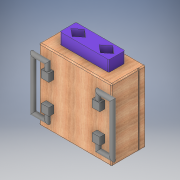
# Autodesk Inventor part: T9 Middle
Saved by Autodesk Inventor 2018 (Build 220112000, 112)
## iProperties
Created: 2018-02-18
Part Number: T9 Middle
Material: Wood (Birch)
Document SubType Name: Modeling
Designer: Blue Mist
Density: 0.55 g/cm^3
Appearance: Birch - Natural Polished
Author: Blue Mist
Autodesk Inventor part; units mm, degrees
ref_plane "YZ Plane" through (0, 0, 0) normal (1, 0, 0) x (0, 1, 0)
ref_plane "XZ Plane" through (0, 0, 0) normal (0, 1, 0) x (-1, 0, 0)
ref_plane "XY Plane" through (0, 0, 0) normal (0, 0, 1) x (1, 0, 0)
sketch "Sketch1" plane through (0, 0, 0) normal (0, 0, 1) x (1, 0, 0)
  line L0 (1.27, 0) -> (80.772, 0)
  line L1 (82.042, 1.27) -> (82.042, 79.375)
  line L2 (80.772, 80.645) -> (1.27, 80.645)
  line L3 (0, 79.375) -> (0, 1.27)
  arc A0 (82.042, 79.375) -> (80.772, 80.645) centre (80.772, 79.375) ccw
  arc A1 (80.772, 0) -> (82.042, 1.27) centre (80.772, 1.27) ccw
  arc A2 (0, 1.27) -> (1.27, 0) centre (1.27, 1.27) ccw
  arc A3 (1.27, 80.645) -> (0, 79.375) centre (1.27, 79.375) ccw
  point P0 (0, 0)
  point P1 (82.042, 80.645)
  point P2 (82.042, 0)
  point P3 (0, 80.645)
  dimension "d0" = 82.042
  dimension "d1" = 80.645
  dimension "d2" = 1.27
  constraints: 8 end point, 8 point on circle, 8 point on line, 8 tangent, 4 centre point, 3 equal radius, 2 parallel, 1 horizontal, 1 perpendicular
  measures "d0" distance of point (0, 80.645) point (82.042, 80.645)
  measures "d1" distance of point (82.042, 80.645) point (82.042, 0)
  measures "d2" radius of A0
extrude "Extrusion1" add sketch "Sketch1" against normal blind 38.5318
sketch "Sketch2" plane through (0, 0, -38.5318) normal (0, 0, -1) x (-1, 0, 0)
  line L0 (-80.772, 0) -> (-1.27, 0) projected
  line L1 (-1.27, 80.645) -> (-80.772, 80.645) projected
  line L2 (0, 1.27) -> (0, 79.375) construction
  line L3 (-82.042, 79.375) -> (-82.042, 1.27) construction
  line L4 (-63.119, 20.8915) -> (-18.923, 20.8915)
  line L5 (-17.653, 22.1615) -> (-17.653, 58.4835)
  line L6 (-18.923, 59.7535) -> (-63.119, 59.7535)
  line L7 (-64.389, 58.4835) -> (-64.389, 22.1615)
  arc A0 (-64.389, 22.1615) -> (-63.119, 20.8915) centre (-63.119, 22.1615) ccw
  arc A1 (-18.923, 20.8915) -> (-17.653, 22.1615) centre (-18.923, 22.1615) ccw
  arc A2 (-17.653, 58.4835) -> (-18.923, 59.7535) centre (-18.923, 58.4835) ccw
  arc A3 (-63.119, 59.7535) -> (-64.389, 58.4835) centre (-63.119, 58.4835) ccw
  point P0 (0, 0)
  point P1 (-64.389, 20.8915)
  point P2 (-17.653, 59.7535)
  dimension "d5" = 80.645
  dimension "d8" = 82.042
  dimension "d9" = 17.653
  dimension "d10" = 20.8915
  dimension "d11" = 20.8915
  dimension "d12" = 17.653
  dimension "d13" = 1.27
  constraints: 8 end point, 8 point on circle, 8 tangent, 4 centre point, 4 point on line, 3 equal radius, 2 parallel, 1 horizontal, 1 perpendicular
  measures "d5" distance between parallel lines of L0 L1
  measures "d8" distance between parallel lines of L2 L3
  measures "d9" distance from line of L3 point (-64.389, 20.892)
  measures "d10" distance from line of L0 point (-64.389, 20.892)
  measures "d11" distance from line of L1 point (-17.653, 59.753)
  measures "d12" distance from line of L2 point (-17.653, 59.753)
  measures "d13" radius of A0
extrude "Extrusion2" cut sketch "Sketch2" against normal blind 29.337
fillet "Fillet1" radius 1.27 16 edges at (81.67, 80.273, -38.5318) (82.042, 40.3225, -38.5318) (81.67, 0.372, -38.5318) (41.021, 0, -38.5318) (0.372, 0.372, -38.5318) (0, 40.3225, -38.5318) (0.372, 80.273, -38.5318) (41.021, 80.645, -38.5318) (81.67, 0.372, 0) (41.021, 0, 0) (0.372, 0.372, 0) (0, 40.3225, 0) (0.372, 80.273, 0) (41.021, 80.645, 0) (81.67, 80.273, 0) (82.042, 40.3225, 0)
sketch "Sketch3" plane through (0, 0, 0) normal (0, 0, 1) x (1, 0, 0)
  line L0 (1.27, 0) -> (80.772, 0) projected
  line L1 (0, 79.375) -> (0, 1.27) projected
  line L2 (80.772, 80.645) -> (1.27, 80.645) projected
  line L3 (82.042, 1.27) -> (82.042, 79.375) projected
  line L4 (74.168, 19.304) -> (65.532, 19.304)
  line L5 (65.532, 19.304) -> (65.532, 27.94)
  line L6 (65.532, 27.94) -> (74.168, 27.94)
  line L7 (74.168, 27.94) -> (74.168, 19.304)
  line L8 (74.168, 61.341) -> (65.532, 61.341)
  line L9 (65.532, 61.341) -> (65.532, 52.705)
  line L10 (65.532, 52.705) -> (74.168, 52.705)
  line L11 (74.168, 52.705) -> (74.168, 61.341)
  line L12 (7.874, 61.341) -> (16.51, 61.341)
  line L13 (16.51, 61.341) -> (16.51, 52.705)
  line L14 (16.51, 52.705) -> (7.874, 52.705)
  line L15 (7.874, 52.705) -> (7.874, 61.341)
  line L16 (7.874, 19.304) -> (16.51, 19.304)
  line L17 (16.51, 19.304) -> (16.51, 27.94)
  line L18 (16.51, 27.94) -> (7.874, 27.94)
  line L19 (7.874, 27.94) -> (7.874, 19.304)
  point P0 (0, 0)
  dimension "d26" = 7.874
  dimension "d27" = 7.874
  dimension "d28" = 7.874
  dimension "d29" = 7.874
  dimension "d30" = 19.304
  dimension "d31" = 19.304
  dimension "d32" = 19.304
  dimension "d33" = 19.304
  dimension "d34" = 8.636
  dimension "d35" = 8.636
  dimension "d36" = 8.636
  dimension "d37" = 8.636
  dimension "d38" = 8.636
  constraints: 32 end point, 8 parallel, 4 horizontal, 4 perpendicular, 3 point on line
  measures "d26" distance from line of L1 L16.start
  measures "d27" distance from line of L1 L12.start
  measures "d28" distance from line of L3 L4.start
  measures "d29" distance from line of L3 L8.start
  measures "d30" distance from line of L2 L8.start
  measures "d31" distance from line of L2 L12.start
  measures "d32" distance from line of L0 L16.start
  measures "d33" distance from line of L0 L4.start
  measures "d34" distance of L5.end L6.end
  measures "d35" distance of L4.end L5.end
  measures "d36" distance of L10.end L9.end
  measures "d37" distance of L9.end L8.end
  measures "d38" distance of L13.end L14.end
extrude "Extrusion3" add sketch "Sketch3" along normal blind 5.461
sketch "Sketch4" plane through (65.532, 61.341, 0) normal (0, 1, 0) x (1, 0, 0)
  line L0 (0, 0) -> (0, -5.461) construction
  line L1 (0, -5.461) -> (8.636, -5.461) construction
  line L2 (8.636, -5.461) -> (0, 0) construction
  line L3 (0, -5.461) -> (8.636, 0) construction
  line L4 (8.636, 0) -> (-49.022, 0) construction
  line L5 (8.636, 0) -> (0, 0) construction
  line L6 (-57.658, 0) -> (-57.658, -5.461) construction
  line L7 (-49.022, 0) -> (-57.658, -5.461) construction
  line L8 (-57.658, -5.461) -> (-49.022, -5.461) construction
  line L9 (-49.022, -5.461) -> (-57.658, 0) construction
  line L10 (-53.34, -2.7305) -> (-53.34, -5.207) construction
  line L11 (-53.34, -5.207) -> (-55.8165, -5.207) construction
  line L12 (-55.8165, -5.207) -> (-50.8635, -5.207)
  line L13 (-50.8635, -5.207) -> (-50.8635, -0.254)
  line L14 (-50.8635, -0.254) -> (-55.8165, -0.254)
  line L15 (-55.8165, -0.254) -> (-55.8165, -5.207)
  line L16 (4.318, -2.7305) -> (4.318, -5.207) construction
  line L17 (4.318, -5.207) -> (1.8415, -5.207) construction
  line L18 (1.8415, -5.207) -> (6.7945, -5.207)
  line L19 (6.7945, -5.207) -> (6.7945, -0.254)
  line L20 (6.7945, -0.254) -> (1.8415, -0.254)
  line L21 (1.8415, -0.254) -> (1.8415, -5.207)
  point P0 (-65.532, 0)
  point P1 (-51.618, -2.9559)
  dimension "d42" = 2.4765
  dimension "d43" = 2.4765
  dimension "d44" = 4.953
  dimension "d45" = 4.953
  dimension "d46" = 2.4765
  dimension "d47" = 2.4765
  dimension "d48" = 4.953
  dimension "d49" = 4.953
  constraints: 36 end point, 6 parallel, 5 perpendicular, 2 horizontal, 2 midpoint, 2 vertical, 1 collinear
  measures "d42" distance of L10.start L10.end
  measures "d43" distance of L10.end L11.end
  measures "d44" distance of L14.end L13.end
  measures "d45" distance of L13.end L12.end
  measures "d46" distance of L16.start L16.end
  measures "d47" distance of L16.end L17.end
  measures "d48" distance of L20.end L19.end
  measures "d49" distance of L19.end L18.end
extrude "Extrusion4" add sketch "Sketch4" along normal blind 10.0965
sketch "Sketch5" plane through (65.532, 19.304, 0) normal (0, -1, 0) x (1, 0, 0)
  line L0 (-55.8165, 5.207) -> (-50.8635, 5.207) projected
  line L1 (-50.8635, 5.207) -> (-50.8635, 0.254) projected
  line L2 (-50.8635, 0.254) -> (-55.8165, 0.254) projected
  line L3 (-55.8165, 0.254) -> (-55.8165, 5.207) projected
  line L4 (1.8415, 5.207) -> (6.7945, 5.207) projected
  line L5 (6.7945, 5.207) -> (6.7945, 0.254) projected
  line L6 (6.7945, 0.254) -> (1.8415, 0.254) projected
  line L7 (1.8415, 0.254) -> (1.8415, 5.207) projected
  point P0 (-65.532, 0)
extrude "Extrusion5" add sketch "Sketch5" along normal blind 10.0965
sketch "Sketch6" plane through (9.7155, 9.2075, 0.254) normal (-1, 0, 0) x (0, 0, 1)
  line L0 (0, 0) -> (4.953, 0) projected
  line L1 (4.953, 10.0965) -> (4.953, 0) projected
  line L2 (0, 0) -> (4.953, 0)
  line L3 (4.953, 0) -> (4.953, 4.953)
  line L4 (4.953, 4.953) -> (0, 4.953)
  line L5 (0, 4.953) -> (0, 0)
  line L6 (4.953, 62.23) -> (0, 62.23) projected
  line L7 (0, 52.1335) -> (0, 62.23) projected
  line L8 (4.953, 62.23) -> (0, 62.23)
  line L9 (0, 62.23) -> (0, 57.277)
  line L10 (0, 57.277) -> (4.953, 57.277)
  line L11 (4.953, 57.277) -> (4.953, 62.23)
  point P0 (-0.254, -9.2075)
  dimension "d54" = 4.953
  dimension "d55" = 4.953
  constraints: 16 end point, 4 parallel, 2 horizontal, 2 perpendicular, 2 point on line
  measures "d54" distance of L3.end L2.end
  measures "d55" distance of L9.end L8.end
extrude "Extrusion6" add sketch "Sketch6" along normal blind 16.002
sketch "Sketch7" plane through (72.3265, 19.304, 5.207) normal (1, 0, 0) x (0, 0, -1)
  line L0 (0, 52.1335) -> (4.953, 52.1335) projected
  line L1 (4.953, 52.1335) -> (4.953, 47.1805) projected
  line L2 (4.953, 47.1805) -> (0, 47.1805) projected
  line L3 (0, 47.1805) -> (0, 52.1335) projected
  line L4 (4.953, -10.0965) -> (0, -10.0965) projected
  line L5 (0, -10.0965) -> (0, -5.1435) projected
  line L6 (0, -5.1435) -> (4.953, -5.1435) projected
  line L7 (4.953, -5.1435) -> (4.953, -10.0965) projected
  point P0 (5.207, -19.304)
extrude "Extrusion7" add sketch "Sketch7" along normal blind 16.002
sketch "Sketch8" plane through (72.3265, 14.1605, 5.207) normal (0, 1, 0) x (1, 0, 0)
  line L0 (0, 0) -> (16.002, 0) projected
  line L1 (16.002, 0) -> (11.049, 0)
  line L2 (11.049, 0) -> (11.049, 4.953)
  line L3 (11.049, 4.953) -> (16.002, 4.953)
  line L4 (16.002, 4.953) -> (16.002, 0)
  line L5 (-78.613, 0) -> (-78.613, 4.953) projected
  line L6 (-78.613, 0) -> (-73.66, 0)
  line L7 (-73.66, 0) -> (-73.66, 4.953)
  line L8 (-73.66, 4.953) -> (-78.613, 4.953)
  line L9 (-78.613, 4.953) -> (-78.613, 0)
  point P0 (-72.3265, 5.207)
  dimension "d60" = 4.953
  dimension "d61" = 4.953
  dimension "d62" = 4.953
  dimension "d63" = 4.953
  constraints: 16 end point, 4 parallel, 2 horizontal, 2 perpendicular
  measures "d60" distance of L2.end L3.end
  measures "d61" distance of L1.end L2.end
  measures "d62" distance of L8.end L7.end
  measures "d63" distance of L7.end L6.end
extrude "Extrusion8" add sketch "Sketch8" along normal through all
fillet "Fillet2" radius 2.4765 40 edges at (88.3285, 40.3225, 5.207) (83.3755, 40.3225, 5.207) (77.851, 14.1605, 5.207) (77.851, 9.2075, 5.207) (77.851, 9.2075, 0.254) (88.3285, 40.3225, 0.254) (77.851, 71.4375, 5.207) (77.851, 71.4375, 0.254) (77.851, 66.4845, 0.254) (77.851, 66.4845, 5.207) (77.851, 14.1605, 0.254) (83.3755, 40.3225, 0.254) (67.3735, 66.3892, 5.207) (72.3265, 63.9127, 5.207) (72.3265, 63.9127, 0.254) (67.3735, 66.3892, 0.254) (67.3735, 14.2558, 0.254) (67.3735, 14.2558, 5.207) (72.3265, 16.7323, 5.207) (72.3265, 16.7323, 0.254) (14.6685, 66.3892, 0.254) (14.6685, 66.3892, 5.207) (4.191, 71.4375, 5.207) (14.6685, 14.2558, 5.207) (14.6685, 14.2558, 0.254) (4.191, 9.2075, 5.207) (4.191, 14.1605, 5.207) (9.7155, 16.7323, 5.207) (-1.3335, 40.3225, 5.207) (-1.3335, 40.3225, 0.254) (-6.2865, 40.3225, 5.207) (4.191, 66.4845, 5.207) (9.7155, 63.9127, 5.207) (-6.2865, 40.3225, 0.254) (4.191, 9.2075, 0.254) (4.191, 14.1605, 0.254) (9.7155, 16.7323, 0.254) (9.7155, 63.9127, 0.254) (4.191, 66.4845, 0.254) (4.191, 71.4375, 0.254)
sketch "Sketch9" plane through (0, 0, -9.1948) normal (0, 0, -1) x (-1, 0, 0)
  line L0 (-64.389, 22.1615) -> (-64.389, 58.4835) construction
  line L1 (-18.923, 20.8915) -> (-63.119, 20.8915) construction
  line L2 (-17.653, 58.4835) -> (-17.653, 22.1615) construction
  line L3 (-63.119, 59.7535) -> (-18.923, 59.7535) construction
  line L4 (-54.229, 30.7975) -> (-27.813, 30.7975) construction
  line L5 (-27.813, 30.7975) -> (-27.813, 49.8475) construction
  line L6 (-27.813, 49.8475) -> (-54.229, 49.8475) construction
  line L7 (-54.229, 49.8475) -> (-54.229, 30.7975) construction
  circle A0 centre (-54.229, 30.7975) radius 7.493
  circle A1 centre (-27.813, 30.7975) radius 7.493
  circle A2 centre (-27.813, 49.8475) radius 7.493
  circle A3 centre (-54.229, 49.8475) radius 7.493
  point P0 (0, 0)
  point P1 (-54.229, 49.8475)
  point P2 (-31.623, 30.7975)
  dimension "d67" = 10.16
  dimension "d68" = 9.906
  dimension "d69" = 9.906
  dimension "d70" = 13.97
  dimension "d71" = 10.16
  dimension "d72" = 9.906
  dimension "d73" = 10.16
  dimension "d74" = 9.906
  dimension "d75" = 14.986
  dimension "d76" = 14.986
  dimension "d77" = 14.986
  dimension "d78" = 14.986
  constraints: 8 end point, 4 centre point, 4 coincident, 2 parallel, 1 horizontal, 1 perpendicular
  measures "d67" distance from line of L0 L4.start
  measures "d68" distance from line of L1 L4.start
  measures "d69" distance from line of L1 point (-31.623, 30.798)
  measures "d70" distance from line of L2 point (-31.623, 30.798)
  measures "d71" distance from line of L2 L5.end
  measures "d72" distance from line of L3 L5.end
  measures "d73" distance from line of L0 point (-54.229, 49.847)
  measures "d74" distance from line of L3 point (-54.229, 49.847)
  measures "d75" diameter of A0
  measures "d76" diameter of A1
  measures "d77" diameter of A2
  measures "d78" diameter of A3
extrude "Extrusion9" cut sketch "Sketch9" against normal blind 7.747
sketch "Sketch10" plane through (1.27, 0, -1.27) normal (0, -1, 0) x (1, 0, 0)
  line L0 (0, -37.2618) -> (79.502, -37.2618) projected
  line L1 (-1.27, 0) -> (-1.27, -35.9918) projected
  line L2 (80.772, 0) -> (80.772, -35.9918) projected
  line L3 (79.502, 1.27) -> (0, 1.27) projected
  line L4 (66.294, -8.763) -> (13.208, -8.763)
  line L5 (11.938, -10.033) -> (11.938, -25.9588)
  line L6 (13.208, -27.2288) -> (66.294, -27.2288)
  line L7 (67.564, -25.9588) -> (67.564, -10.033)
  arc A0 (11.938, -25.9588) -> (13.208, -27.2288) centre (13.208, -25.9588) ccw
  arc A1 (13.208, -8.763) -> (11.938, -10.033) centre (13.208, -10.033) ccw
  arc A2 (67.564, -10.033) -> (66.294, -8.763) centre (66.294, -10.033) ccw
  arc A3 (66.294, -27.2288) -> (67.564, -25.9588) centre (66.294, -25.9588) ccw
  point P0 (-1.27, 1.27)
  point P1 (11.938, -27.2288)
  point P2 (67.564, -8.763)
  dimension "d81" = 10.033
  dimension "d82" = 13.208
  dimension "d83" = 13.208
  dimension "d84" = 10.033
  dimension "d85" = 1.27
  constraints: 8 end point, 8 point on circle, 8 tangent, 4 centre point, 4 point on line, 3 equal radius, 2 parallel, 1 horizontal, 1 perpendicular
  measures "d81" distance from line of point (11.938, -27.229) L0
  measures "d82" distance from line of L1 point (11.938, -27.229)
  measures "d83" distance from line of L2 point (67.564, -8.763)
  measures "d84" distance from line of L3 point (67.564, -8.763)
  measures "d85" radius of A0
extrude "Extrusion10" cut sketch "Sketch10" against normal blind 12.573
sketch "Sketch11" plane through (1.27, 12.573, -1.27) normal (0, -1, 0) x (1, 0, 0)
  line L0 (66.294, -27.2288) -> (13.208, -27.2288) projected
  line L1 (13.208, -8.763) -> (66.294, -8.763) projected
  line L2 (67.564, -10.033) -> (67.564, -25.9588) projected
  line L3 (64.008, -17.9959) -> (55.753, -11.176)
  line L4 (55.753, -11.176) -> (47.498, -17.9959)
  line L5 (47.498, -17.9959) -> (55.753, -24.8158)
  line L6 (55.753, -24.8158) -> (64.008, -17.9959)
  line L7 (11.938, -25.9588) -> (11.938, -10.033) projected
  line L8 (23.749, -24.8158) -> (32.004, -17.9959)
  line L9 (32.004, -17.9959) -> (23.749, -11.176)
  line L10 (23.749, -11.176) -> (15.494, -17.9959)
  line L11 (15.494, -17.9959) -> (23.749, -24.8158)
  point P0 (-1.27, 1.27)
  point P1 (55.753, -17.9959)
  point P2 (23.749, -17.9959)
  dimension "d88" = 9.2329
  dimension "d89" = 18.4658
  dimension "d90" = 3.556
  dimension "d91" = 16.51
  dimension "d92" = 8.255
  dimension "d93" = 2.413
  dimension "d94" = 2.413
  dimension "d95" = 3.556
  dimension "d96" = 16.51
  dimension "d97" = 8.255
  constraints: 16 end point, 4 parallel, 1 point on line
  measures "d88" distance from line of L0 L3.start
  measures "d89" distance between parallel lines of L1 L0
  measures "d90" distance from line of L2 L3.start
  measures "d91" distance of L4.end L3.start
  measures "d92" distance of L4.end point (55.753, -17.996)
  measures "d93" distance from line of L0 L5.end
  measures "d94" distance from line of L1 L3.end
  measures "d95" distance from line of L7 L10.end
  measures "d96" distance of L10.end L8.end
  measures "d97" distance of L8.end point (23.749, -17.996)
extrude "Extrusion11" add sketch "Sketch11" along normal blind 12.573
sketch "Sketch12" plane through (1.27, 80.645, -1.27) normal (0, 1, 0) x (1, 0, 0)
  line L0 (23.749, 11.176) -> (15.494, 17.9959) projected
  line L1 (15.494, 17.9959) -> (23.749, 24.8158) projected
  line L2 (23.749, 24.8158) -> (32.004, 17.9959) projected
  line L3 (32.004, 17.9959) -> (23.749, 11.176) projected
  line L4 (64.008, 17.9959) -> (55.753, 11.176) projected
  line L5 (55.753, 11.176) -> (47.498, 17.9959) projected
  line L6 (47.498, 17.9959) -> (55.753, 24.8158) projected
  line L7 (55.753, 24.8158) -> (64.008, 17.9959) projected
  line L8 (64.008, 17.9959) -> (55.753, 24.8158) projected
  line L9 (55.753, 24.8158) -> (47.498, 17.9959) projected
  line L10 (47.498, 17.9959) -> (55.753, 11.176) projected
  line L11 (55.753, 11.176) -> (64.008, 17.9959) projected
  line L12 (23.749, 11.176) -> (32.004, 17.9959) projected
  line L13 (32.004, 17.9959) -> (23.749, 24.8158) projected
  line L14 (23.749, 24.8158) -> (15.494, 17.9959) projected
  line L15 (15.494, 17.9959) -> (23.749, 11.176) projected
  line L16 (11.938, 25.9588) -> (11.938, 10.033) projected
  arc A0 (13.208, 27.2288) -> (11.938, 25.9588) centre (13.208, 25.9588) ccw projected
  line L17 (66.294, 27.2288) -> (13.208, 27.2288) projected
  arc A1 (67.564, 25.9588) -> (66.294, 27.2288) centre (66.294, 25.9588) ccw projected
  line L18 (67.564, 10.033) -> (67.564, 25.9588) projected
  arc A2 (66.294, 8.763) -> (67.564, 10.033) centre (66.294, 10.033) ccw projected
  line L19 (13.208, 8.763) -> (66.294, 8.763) projected
  arc A3 (11.938, 10.033) -> (13.208, 8.763) centre (13.208, 10.033) ccw projected
  point P0 (-1.27, -1.27)
extrude "Extrusion12" add sketch "Sketch12" along normal blind 12.573
sketch "Sketch13" plane through (0, 1.27, -1.27) normal (-1, 0, 0) x (0, 0, 1)
  line L0 (-37.2618, 78.105) -> (-37.2618, 0) projected
  line L1 (-30.48, 15.8063) -> (-30.48, 79.375)
  line L2 (-28.702, 15.8063) -> (-28.702, 79.375)
  line L3 (0, 79.375) -> (-35.9918, 79.375) projected
  line L4 (-28.702, 15.8063) -> (-28.702, -1.27)
  line L5 (-27.2288, -1.27) -> (-27.2288, 11.303) projected
  line L6 (-30.48, 15.8063) -> (-30.48, -1.27)
  line L7 (0, -1.27) -> (-35.9918, -1.27) projected
  line L8 (-28.702, -1.27) -> (-30.48, -1.27)
  line L9 (-30.48, 79.375) -> (-28.702, 79.375)
  point P0 (1.27, -1.27)
  dimension "d102" = 6.7818
  dimension "d103" = 1.778
  constraints: 12 end point, 3 vertical, 2 point on line, 1 collinear, 1 parallel, 1 perpendicular
  measures "d102" distance from line of L0 L1.start
  measures "d103" distance of L1.start L2.start
extrude "Extrusion13" cut sketch "Sketch13" against normal blind 1.27
sketch "Sketch14" plane through (82.042, 1.27, -1.27) normal (1, 0, 0) x (0, 0, -1)
  line L0 (30.48, 0) -> (30.48, 78.105) projected
  line L1 (28.702, 78.105) -> (28.702, 0) projected
  line L2 (30.48, 78.105) -> (30.48, 79.375) projected
  line L3 (30.48, 78.105) -> (30.48, 79.375)
  line L4 (30.48, 79.375) -> (28.702, 79.375)
  line L5 (0, 79.375) -> (35.9918, 79.375) projected
  line L6 (0, 79.375) -> (28.702, 79.375) projected
  line L7 (28.702, 78.105) -> (28.702, 79.375)
  line L8 (30.48, 0) -> (30.48, -1.27)
  line L9 (0, -1.27) -> (35.9918, -1.27) projected
  line L10 (28.702, -1.27) -> (28.702, 0)
  line L11 (28.702, -1.27) -> (30.48, -1.27)
  line L12 (0, -1.27) -> (28.702, -1.27) projected
  point P0 (-1.27, -1.27)
  constraints: 12 end point, 2 point on line, 2 vertical, 1 collinear, 1 parallel, 1 perpendicular
extrude "Extrusion14" cut sketch "Sketch14" against normal blind 1.27
sketch "Sketch15" plane through (1.27, 93.218, -1.27) normal (0, 1, 0) x (1, 0, 0)
  line L0 (80.772, 0) -> (80.772, 28.702) projected
  line L1 (67.564, 10.033) -> (67.564, 25.9588) projected
  line L2 (-1.27, 0) -> (-1.27, 28.702) projected
  line L3 (11.938, 25.9588) -> (11.938, 10.033) projected
  line L4 (79.502, 37.2618) -> (0, 37.2618) projected
  line L5 (66.294, 27.2288) -> (13.208, 27.2288) projected
  line L6 (0, -1.27) -> (79.502, -1.27) projected
  line L7 (13.208, 8.763) -> (66.294, 8.763) projected
  line L8 (55.753, 11.176) -> (47.498, 17.9959) projected
  line L9 (47.498, 17.9959) -> (55.753, 24.8158) projected
  line L10 (55.753, 24.8158) -> (64.008, 17.9959) projected
  line L11 (64.008, 17.9959) -> (55.753, 11.176) projected
  line L12 (15.494, 17.9959) -> (23.749, 24.8158) projected
  line L13 (23.749, 24.8158) -> (32.004, 17.9959) projected
  line L14 (32.004, 17.9959) -> (23.749, 11.176) projected
  line L15 (23.749, 11.176) -> (15.494, 17.9959) projected
  line L16 (11.938, 25.9588) -> (11.938, 10.033) projected
  arc A0 (11.938, 10.033) -> (13.208, 8.763) centre (13.208, 10.033) ccw projected
  line L17 (13.208, 8.763) -> (66.294, 8.763) projected
  arc A1 (66.294, 8.763) -> (67.564, 10.033) centre (66.294, 10.033) ccw projected
  line L18 (67.564, 10.033) -> (67.564, 25.9588) projected
  arc A2 (67.564, 25.9588) -> (66.294, 27.2288) centre (66.294, 25.9588) ccw projected
  line L19 (66.294, 27.2288) -> (13.208, 27.2288) projected
  arc A3 (13.208, 27.2288) -> (11.938, 25.9588) centre (13.208, 25.9588) ccw projected
  line L20 (39.0635, 8.89) -> (47.9125, 8.89) construction
  line L21 (47.9125, 8.89) -> (73.2045, 8.89) construction
  line L22 (73.2045, 8.89) -> (7.0483, 8.89) construction
  line L23 (12.065, 20.82) -> (12.065, 16.1073) construction
  line L24 (12.065, 16.1073) -> (12.065, 4.938) construction
  line L25 (12.065, 4.938) -> (12.065, 30.0903) construction
  line L26 (35.4412, 27.1018) -> (40.4206, 27.1018) construction
  line L27 (40.4206, 27.1018) -> (70.8788, 27.1018) construction
  line L28 (47.498, 17.9959) -> (55.753, 24.8158) construction
  line L29 (50.7658, 20.8603) -> (52.4476, 22.2498) construction
  line L30 (52.4476, 22.2498) -> (60.2576, 28.702) construction
  line L31 (60.2576, 28.702) -> (46.5047, 17.34) construction
  line L32 (67.564, 10.033) -> (67.564, 25.9588) construction
  line L33 (67.437, 19.8845) -> (67.437, 16.1073) construction
  line L34 (67.437, 16.1073) -> (67.437, 6.2841) construction
  line L35 (67.437, 16.1073) -> (67.437, 19.8845) construction
  line L36 (58.4038, 22.7906) -> (60.598, 20.9778) construction
  line L37 (60.598, 20.9778) -> (65.2544, 17.1309) construction
  line L38 (65.2544, 17.1309) -> (54.5689, 25.9588) construction
  line L39 (57.8734, 12.763) -> (59.9614, 14.488) construction
  line L40 (59.9614, 14.488) -> (66.1615, 19.6103) construction
  line L41 (66.1615, 19.6103) -> (54.5689, 10.033) construction
  line L42 (50.9965, 14.9408) -> (53.1022, 13.2012) construction
  line L43 (53.1022, 13.2012) -> (57.8734, 9.2595) construction
  line L44 (57.8734, 9.2595) -> (46.0174, 19.0543) construction
  line L45 (19.038, 14.9032) -> (20.5442, 13.6589) construction
  line L46 (20.5442, 13.6589) -> (25.5018, 9.5632) construction
  line L47 (25.5018, 9.5632) -> (14.2589, 18.8516) construction
  line L48 (23.749, 24.8158) -> (15.494, 17.9959) construction
  line L49 (18.3706, 20.5372) -> (21.0982, 22.7906) construction
  line L50 (21.0982, 22.7906) -> (24.3486, 25.4759) construction
  line L51 (24.3486, 25.4759) -> (13.495, 16.5091) construction
  line L52 (27.9574, 21.5038) -> (29.6383, 20.1151) construction
  line L53 (29.6383, 20.1151) -> (33.2504, 17.1309) construction
  line L54 (33.2504, 17.1309) -> (23.3203, 25.3347) construction
  line L55 (29.0748, 15.4112) -> (26.7291, 13.4733) construction
  line L56 (26.7291, 13.4733) -> (22.5649, 10.033) construction
  line L57 (22.5649, 10.033) -> (33.6992, 19.2317) construction
  line L58 (13.335, 8.89) -> (66.167, 8.89)
  line L59 (67.437, 10.16) -> (67.437, 25.8318)
  line L60 (66.167, 27.1018) -> (13.335, 27.1018)
  line L61 (12.065, 25.8318) -> (12.065, 10.16)
  arc A4 (12.065, 10.16) -> (13.335, 8.89) centre (13.335, 10.16) ccw
  arc A5 (66.167, 8.89) -> (67.437, 10.16) centre (66.167, 10.16) ccw
  arc A6 (13.335, 27.1018) -> (12.065, 25.8318) centre (13.335, 25.8318) ccw
  arc A7 (67.437, 25.8318) -> (66.167, 27.1018) centre (66.167, 25.8318) ccw
  line L62 (15.2946, 17.9959) -> (23.749, 24.9805)
  line L63 (32.2034, 17.9959) -> (23.749, 24.9805)
  line L64 (32.2034, 17.9959) -> (23.749, 11.0113)
  line L65 (23.749, 11.0113) -> (15.2946, 17.9959)
  line L66 (47.2986, 17.9959) -> (55.753, 11.0113)
  line L67 (55.753, 11.0113) -> (64.2074, 17.9959)
  line L68 (64.2074, 17.9959) -> (55.753, 24.9805)
  line L69 (64.008, 17.9959) -> (55.753, 24.8158) projected
  line L70 (47.2986, 17.9959) -> (55.753, 24.9805)
  point P0 (-1.27, -1.27)
  point P1 (12.065, 8.89)
  point P2 (12.065, 27.1018)
  point P3 (67.437, 8.89)
  dimension "d108" = 13.208
  dimension "d109" = 13.208
  dimension "d110" = 10.033
  dimension "d111" = 10.033
  dimension "d112" = 0.127
  dimension "d113" = 0.127
  dimension "d114" = 0.127
  dimension "d115" = 0.127
  dimension "d116" = 0.127
  dimension "d117" = 0.127
  dimension "d118" = 0.127
  dimension "d119" = 0.127
  dimension "d120" = 0.127
  dimension "d121" = 0.127
  dimension "d122" = 0.127
  dimension "d123" = 0.127
  dimension "d124" = 0.127
  dimension "d125" = 0.127
  dimension "d126" = 0.127
  dimension "d127" = 0.127
  dimension "d128" = 0.127
  dimension "d129" = 0.127
  dimension "d130" = 0.127
  dimension "d131" = 0.127
  dimension "d132" = 0.127
  dimension "d133" = 0.127
  dimension "d134" = 0.127
  dimension "d135" = 0.127
  dimension "d136" = 180
  dimension "d137" = 180
  dimension "d138" = 180
  dimension "d139" = 180
  dimension "d140" = 0
  dimension "d141" = 180
  dimension "d142" = 0
  dimension "d143" = 1.27
  dimension "d144" = 1.27
  dimension "d145" = 1.27
  constraints: 94 end point, 39 point on line, 8 point on circle, 8 tangent, 5 parallel, 4 centre point, 2 collinear, 1 equal radius, 1 horizontal, 1 perpendicular
  measures "d108" distance between parallel lines of L0 L1
  measures "d109" distance between parallel lines of L2 L3
  measures "d110" distance between parallel lines of L4 L5
  measures "d111" distance between parallel lines of L6 L7
  measures "d112" distance from line of L3 L23.end
  measures "d113" distance from line of L3 L23.start
  measures "d114" distance from line of L15 L45.start
  measures "d115" distance from line of L15 L45.end
  measures "d116" distance from line of L14 L55.end
  measures "d117" distance from line of L14 L55.start
  measures "d118" distance from line of L13 L52.end
  measures "d119" distance from line of L13 L52.start
  measures "d120" distance from line of L12 L49.end
  measures "d121" distance from line of L12 L49.start
  measures "d122" distance from line of L19 L26.start
  measures "d123" distance from line of L19 L26.end
  measures "d124" distance from line of L17 L20.start
  measures "d125" distance from line of L17 L20.end
  measures "d126" distance from line of L42.end L8
  measures "d127" distance from line of L8 L42.start
  measures "d128" distance from line of L9 L29.start
  measures "d129" distance from line of L9 L29.end
  measures "d130" distance from line of L10 L36.start
  measures "d131" distance from line of L10 L36.end
  measures "d132" distance from line of L11 L39.end
  measures "d133" distance from line of L11 L39.start
  measures "d134" distance from line of L1 L33.end
  measures "d135" distance from line of L1 L33.start
  measures "d136" angle of L20 L21
  measures "d137" angle of L27 L26
  measures "d138" angle of L30 L29
  measures "d139" angle of L37 L36
  measures "d140" distance between parallel lines of L38 L37
  measures "d141" angle of L40 L39
  measures "d142" distance between parallel lines of L41 L40
  measures "d143" radius of A4
  measures "d144" radius of A6
  measures "d145" radius of A7
extrude "Extrusion15" cut sketch "Sketch15" against normal blind 12.573
sketch "Sketch16" plane through (0, 0, -38.5318) normal (0, 0, -1) x (-1, 0, 0)
  line L0 (-17.653, 58.4835) -> (-17.653, 22.1615) projected
  line L1 (-63.119, 59.7535) -> (-18.923, 59.7535) projected
  line L2 (-64.389, 22.1615) -> (-64.389, 58.4835) projected
  line L3 (-18.923, 20.8915) -> (-63.119, 20.8915) projected
  arc A0 (-17.653, 58.4835) -> (-18.923, 59.7535) centre (-18.923, 58.4835) ccw projected
  arc A1 (-63.119, 59.7535) -> (-64.389, 58.4835) centre (-63.119, 58.4835) ccw projected
  arc A2 (-64.389, 22.1615) -> (-63.119, 20.8915) centre (-63.119, 22.1615) ccw projected
  arc A3 (-18.923, 20.8915) -> (-17.653, 22.1615) centre (-18.923, 22.1615) ccw projected
  line L4 (-17.526, 30.9752) -> (-17.526, 54.1428) construction
  line L5 (-17.526, 30.9752) -> (-17.526, 61.341) construction
  line L6 (-16.51, 61.341) -> (-16.51, 52.705) construction
  line L7 (-30.618, 20.7645) -> (-57.868, 20.7645) construction
  line L8 (-57.868, 20.7645) -> (-70.0448, 20.7645) construction
  line L9 (-64.516, 34.8535) -> (-64.516, 54.1428) construction
  line L10 (-54.1939, 59.8805) -> (-32.4551, 59.8805) construction
  line L11 (-32.4551, 59.8805) -> (-9.5378, 59.8805) construction
  line L12 (-18.796, 20.7645) -> (-63.246, 20.7645)
  line L13 (-64.516, 22.0345) -> (-64.516, 58.6105)
  line L14 (-63.246, 59.8805) -> (-18.796, 59.8805)
  line L15 (-17.526, 58.6105) -> (-17.526, 22.0345)
  arc A4 (-63.246, 59.8805) -> (-64.516, 58.6105) centre (-63.246, 58.6105) ccw
  arc A5 (-17.526, 58.6105) -> (-18.796, 59.8805) centre (-18.796, 58.6105) ccw
  arc A6 (-64.516, 22.0345) -> (-63.246, 20.7645) centre (-63.246, 22.0345) ccw
  arc A7 (-18.796, 20.7645) -> (-17.526, 22.0345) centre (-18.796, 22.0345) ccw
  point P0 (0, 0)
  point P1 (-17.526, 59.8805)
  point P2 (-64.516, 20.7645)
  dimension "d148" = 0.127
  dimension "d149" = 0.127
  dimension "d150" = 0.127
  dimension "d151" = 0.127
  dimension "d152" = 0.127
  dimension "d153" = 0.127
  dimension "d154" = 0.127
  dimension "d155" = 0.127
  dimension "d156" = 180
  dimension "d157" = 1.27
  dimension "d158" = 1.27
  constraints: 22 end point, 8 point on circle, 8 tangent, 4 centre point, 3 parallel, 2 equal radius, 1 horizontal, 1 perpendicular, 1 point on line
  measures "d148" distance from line of L0 L4.start
  measures "d149" distance from line of L0 L4.end
  measures "d150" distance from line of L1 L10.end
  measures "d151" distance from line of L1 L10.start
  measures "d152" distance from line of L2 L9.end
  measures "d153" distance from line of L2 L9.start
  measures "d154" distance from line of L3 L7.end
  measures "d155" distance from line of L3 L7.start
  measures "d156" angle of L8 L7
  measures "d157" radius of A4
  measures "d158" radius of A7
extrude "Extrusion16" cut sketch "Sketch16" against normal blind 29.337
body "Solid1"
